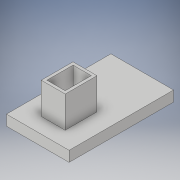
# Autodesk Inventor part: main_chassis
Saved by Autodesk Inventor 2017 (Build 210142000, 142)
## iProperties
Created: 2016-08-29
Part Number: main_chassis
Material: Generic
Document SubType Name: Modeling
Designer: yash
Density: 1 g/cm^3
Appearance: Default
Author: yash
Autodesk Inventor part; units mm, degrees
ref_plane "YZ Plane" through (0, 0, 0) normal (1, 0, 0) x (0, 1, 0)
ref_plane "XZ Plane" through (0, 0, 0) normal (0, 1, 0) x (-1, 0, 0)
ref_plane "XY Plane" through (0, 0, 0) normal (0, 0, 1) x (1, 0, 0)
sketch "Sketch1" plane through (0, 0, 0) normal (0, 0, 1) x (1, 0, 0)
  line L0 (0, 0) -> (38.1, 0)
  line L1 (38.1, 0) -> (38.1, 6.35)
  line L2 (38.1, 6.35) -> (0, 6.35)
  line L3 (0, 6.35) -> (0, 0)
  line L4 (1.7272, 5.4864) -> (36.3728, 5.4864)
  line L5 (36.3728, 5.4864) -> (36.3728, 0.8636)
  line L6 (36.3728, 0.8636) -> (1.7272, 0.8636)
  line L7 (1.7272, 0.8636) -> (1.7272, 5.4864)
  dimension "d0" = 38.1
  dimension "d1" = 6.35
  dimension "d2" = 0.8636
  dimension "d3" = 1.7272
  dimension "d4" = 0.8636
  dimension "d5" = 1.7272
  constraints: 16 end point, 4 parallel, 2 horizontal, 2 perpendicular
  measures "d0" distance of L2.end L1.end
  measures "d1" distance of L1.end L0.end
  measures "d2" distance between parallel lines of L2 L4
  measures "d3" distance between parallel lines of L3 L7
  measures "d4" distance between parallel lines of L0 L6
  measures "d5" distance between parallel lines of L1 L5
extrude "Extrusion1" add sketch "Sketch1" along normal blind 63.5
sketch "Sketch2" plane through (0, 0, 0) normal (0, -1, 0) x (1, 0, 0)
  line L0 (0, 63.5) -> (38.1, 63.5) projected
  circle A0 centre (19.05, 44.45) radius 16.51
  point P0 (0, 0)
  point P1 (19.05, 63.5)
  point P2 (19.05, 63.5)
  dimension "d8" = 33.02
  dimension "d9" = 19.05
  constraints: 2 midpoint, 1 centre point, 1 vertical alignment
  measures "d8" diameter of A0
  measures "d9" distance of point (19.05, 63.5) A0.centre
extrude "Extrusion2" cut sketch "Sketch2" against normal up to next
sketch "Sketch3" plane through (1.7272, 5.4864, 0) normal (0, -1, 0) x (1, 0, 0)
  circle A0 centre (17.3228, 44.45) radius 16.51 construction
  line L0 (36.3728, 63.5) -> (-1.7272, 63.5) construction
  arc A1 (0, 44.45) -> (17.3228, 27.1272) centre (17.3228, 44.45) ccw
  line L1 (17.3228, 44.45) -> (0, 44.45) construction
  line L2 (17.3228, 44.45) -> (34.6456, 44.45) construction
  line L3 (17.3228, 44.45) -> (17.3228, 27.1272) construction
  line L4 (-1.7272, 0) -> (-1.7272, 63.5) projected
  arc A2 (17.3228, 27.1272) -> (0, 9.8044) centre (17.3228, 9.8044) ccw
  line L5 (17.3228, 9.8044) -> (0, 9.8044) construction
  line L6 (17.3228, 9.8044) -> (17.3228, 27.1272) construction
  arc A3 (34.6456, 44.45) -> (0, 44.45) centre (17.3228, 44.45) ccw
  line L7 (34.6456, 44.45) -> (34.6456, 61.7728)
  line L8 (34.6456, 61.7728) -> (0, 61.7728)
  line L9 (0, 61.7728) -> (0, 9.8044)
  point P0 (17.3228, 63.5)
  point P1 (17.3228, 61.7728)
  dimension "d12" = 33.02
  dimension "d13" = 19.05
  dimension "d14" = 180
  dimension "d15" = 90
  dimension "d16" = 1.7272
  dimension "d17" = 90
  dimension "d19" = 1.7272
  dimension "d20" = 19.05
  constraints: 16 end point, 7 point on circle, 4 centre point, 2 coincident, 2 midpoint, 2 perpendicular, 2 vertical alignment, 1 collinear, 1 horizontal, 1 tangent, 1 vertical
  measures "d12" diameter of A0
  measures "d13" distance of point (17.323, 63.5) A0.centre
  measures "d14" angle of L1 L2
  measures "d15" angle of L1 L3
  measures "d16" distance from line of L4 L1.end
  measures "d17" angle of L6 L5
  measures "d19" distance between parallel lines of L0 L8
  measures "d20" distance from line of A1.start L0
extrude "Extrusion4" add sketch "Sketch3" along normal up to next contours L8 L7 A3
sketch "Sketch5" plane through (1.7272, 5.4864, 63.5) normal (0, -1, 0) x (1, 0, 0)
  arc A0 (17.3228, -1.7272) -> (0, -19.05) centre (17.3228, -19.05) ccw
  line L0 (17.3228, -19.05) -> (0, -19.05) construction
  line L1 (17.3228, -19.05) -> (17.3228, -1.7272) construction
  line L2 (36.3728, 0) -> (-1.7272, 0) construction
  line L3 (-1.7272, -63.5) -> (-1.7272, 0) construction
  line L4 (17.3228, -1.7272) -> (0, -1.7272)
  line L5 (0, -1.7272) -> (0, -19.05)
  point P0 (17.3228, 0)
  dimension "d35" = 90
  dimension "d36" = 1.7272
  dimension "d37" = 1.7272
  constraints: 8 end point, 2 point on circle, 1 centre point, 1 horizontal, 1 midpoint, 1 perpendicular, 1 tangent, 1 vertical alignment
  measures "d35" angle of L1 L0
  measures "d36" distance of point (17.323, 0) L1.end
  measures "d37" distance from line of L0.end L3
extrude "Extrusion5" add sketch "Sketch5" along normal up to next
sketch "Sketch6" plane through (1.7272, 5.4864, 0) normal (0, -1, 0) x (1, 0, 0)
  arc A0 (0, 44.45) -> (17.3228, 27.1272) centre (17.3228, 44.45) ccw
  line L0 (17.3228, 44.45) -> (17.3228, 27.1272) construction
  line L1 (17.3228, 44.45) -> (0, 44.45) construction
  line L2 (36.3728, 63.5) -> (-1.7272, 63.5) projected
  line L3 (-1.7272, 0) -> (-1.7272, 63.5) projected
  line L4 (17.3228, 9.8044) -> (0, 9.8044) construction
  line L5 (17.3228, 9.8044) -> (17.3228, 27.1272) construction
  line L6 (0, 44.45) -> (0, 9.8044)
  line L7 (17.3228, 27.1272) -> (0, 9.8044)
  point P0 (17.3228, 63.5)
  dimension "d40" = 90
  dimension "d41" = 1.7272
  dimension "d42" = 19.05
  dimension "d43" = 90
  dimension "d44" = 1.7272
  dimension "d45" = 17.3228
  constraints: 12 end point, 2 point on circle, 2 vertical alignment, 1 centre point, 1 midpoint, 1 parallel
  measures "d40" angle of L1 L0
  measures "d41" distance from line of L3 L1.end
  measures "d42" distance from line of L2 L0.start
  measures "d43" angle of L5 L4
  measures "d44" distance from line of L3 L4.end
  measures "d45" horizontal distance of L0.end L4.end
extrude "Extrusion6" add sketch "Sketch6" along normal up to next
sketch "Sketch7" plane through (1.7272, 5.4864, 61.7728) normal (0, 0, 1) x (1, 0, 0)
  line L0 (17.3228, -4.6228) -> (0, -4.6228) projected
  line L1 (17.3228, 0) -> (34.6456, 0) projected
  line L2 (0, -4.6228) -> (34.6456, -4.6228)
  line L3 (34.6456, -4.6228) -> (34.6456, 0)
  line L4 (34.6456, 0) -> (0, 0)
  line L5 (0, 0) -> (0, -4.6228)
  point P0 (-1.7272, -5.4864)
  constraints: 8 end point, 2 parallel, 1 horizontal, 1 perpendicular
extrude "Extrusion7" add sketch "Sketch7" along normal blind 1.7272
sketch "Sketch8" plane through (0, 6.35, 0) normal (0, 1, 0) x (1, 0, 0)
  line L0 (38.1, -63.5) -> (0, -63.5) projected
  line L1 (13.4938, -52.3875) -> (24.6062, -52.3875)
  line L2 (24.6062, -52.3875) -> (24.6062, -36.5125)
  line L3 (24.6062, -36.5125) -> (13.4938, -36.5125)
  line L4 (13.4938, -36.5125) -> (13.4938, -52.3875)
  line L5 (11.7666, -54.1147) -> (26.3335, -54.1147)
  line L6 (26.3335, -54.1147) -> (26.3335, -34.7853)
  line L7 (26.3335, -34.7853) -> (11.7665, -34.7853)
  line L8 (11.7665, -34.7853) -> (11.7666, -54.1147)
  point P0 (0, 0)
  point P1 (19.05, -44.45)
  point P2 (19.05, -63.5)
  point P3 (19.05, -36.5125)
  point P4 (13.4937, -44.45)
  dimension "d50" = 19.05
  dimension "d51" = 11.1125
  dimension "d52" = 15.875
  dimension "d53" = 1.7272
  dimension "d54" = 1.7272
  dimension "d55" = 1.7272
  dimension "d56" = 1.7272
  constraints: 16 end point, 4 parallel, 3 midpoint, 2 horizontal, 2 perpendicular, 2 vertical alignment, 1 horizontal alignment
  measures "d50" distance from line of L0 point (19.05, -44.45)
  measures "d51" distance of L2.end L3.end
  measures "d52" distance of L3.end L1.start
  measures "d53" distance between parallel lines of L6 L2
  measures "d54" distance between parallel lines of L5 L1
  measures "d55" distance between parallel lines of L4 L8
  measures "d56" distance between parallel lines of L3 L7
extrude "Extrusion8" add sketch "Sketch8" along normal blind 19.05
sketch "Sketch9" plane through (0, 6.35, 0) normal (0, 1, 0) x (1, 0, 0)
  line L0 (38.1, -63.5) -> (0, -63.5) projected
  line L1 (13.4938, -52.3875) -> (13.4938, -36.5125) projected
  point P0 (0, 0)
  point P1 (19.05, -44.45)
  point P2 (19.05, -63.5)
  point P3 (13.4938, -44.45)
  constraints: 2 midpoint, 1 horizontal alignment, 1 vertical alignment
hole "Hole1" at (19.05, 6.35, 44.45) direction (0, -1, 0) diameter 4.7625 end through all
body "Solid1"
